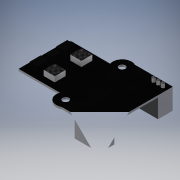
# Autodesk Inventor part: Encoder
Saved by Autodesk Inventor 2016 (Build 200138000, 138)
## iProperties
Created: 2017-02-27
Part Number: Encoder
Material: Generic
Document SubType Name: Modeling
Designer: jorge
Density: 1 g/cm^3
Appearance: Gray
Author: jorge
Autodesk Inventor part; units mm, degrees
note: some values were not read from the file. Chosen so that the rebuilt part matches the saved one: sketch regions of "Extrusion1".
ref_plane "YZ Plane" through (0, 0, 0) normal (1, 0, 0) x (0, 1, 0)
ref_plane "XZ Plane" through (0, 0, 0) normal (0, 1, 0) x (-1, 0, 0)
ref_plane "XY Plane" through (0, 0, 0) normal (0, 0, 1) x (1, 0, 0)
sketch "Sketch1" plane through (0, 0, 0) normal (0, 1, 0) x (-1, 0, 0)
  line L0 (0, 0) -> (0, -16)
  line L1 (0, -16) -> (-13, -16)
  circle A0 centre (48.4003, -12.7173) radius 1 projected
  circle A1 centre (48.4003, 5.2827) radius 1 projected
  line L2 (0, 0) -> (-13, 0)
  line L3 (-16, 0) -> (-16, 1.0033)
  line L4 (-16, -16) -> (-16, -17.0033)
  circle A2 centre (-16, 1.0033) radius 1
  circle A3 centre (-16, -17.0033) radius 1
  arc A4 (-18.8273, -16) -> (-13.1727, -16) centre (-16, -17.0033) ccw
  arc A5 (-13.1727, 0) -> (-18.8273, 0) centre (-16, 1.0033) ccw
  line L5 (-19, 0) -> (-29.5, 0)
  line L6 (-19, -16) -> (-29.5, -16)
  line L7 (-29.5, 0) -> (-29.5, -16)
  line L8 (-29.5, -8) -> (-29.5, -19.65)
  line L9 (-29.5, -8) -> (-29.5, 3.6592)
  line L10 (-29.5, 3.6592) -> (-17.3951, 3.6592)
  line L11 (-29.5, -19.65) -> (-17.4124, -19.65)
  line L12 (-13, 0) -> (-13.1727, 0)
  line L13 (-18.8273, 0) -> (-19, 0)
  line L14 (-13, -16) -> (-13.1727, -16)
  line L15 (-18.8273, -16) -> (-19, -16)
  dimension "d0" = 16
  dimension "d1" = 13
  dimension "d2" = 6
  dimension "d3" = 1.0033
  dimension "d4" = 1.0033
  dimension "d5" = 2
  dimension "d6" = 2
  dimension "d7" = 6
  dimension "d8" = 6
  dimension "d9" = 6
  dimension "d10" = 13
  dimension "d11" = 10.5
  dimension "d12" = 11.65
  constraints: 32 end point, 6 horizontal, 6 point on circle, 5 vertical, 4 centre point, 4 coincident, 2 point on line, 1 midpoint, 1 parallel, 1 perpendicular
  measures "d0" distance of L0.start L0.end
  measures "d1" distance of L0.end L1.end
  measures "d2" distance of L2.end L5.start
  measures "d3" distance of L3.start L3.end
  measures "d4" distance of L4.start L4.end
  measures "d5" diameter of A2
  measures "d6" diameter of A3
  measures "d7" diameter of A4
  measures "d8" diameter of A5
  measures "d9" distance of L1.end L6.start
  measures "d10" distance of L0.start L2.end
  measures "d11" distance of L5.start L5.end
  measures "d12" distance of L8.start L8.end
extrude "Extrusion1" add sketch "Sketch1" along normal blind 0.65 contours L0 L1 L14 A4 L15 L6 L7 L5 L13 A5 L12 L2 | A5 L13 L5 L9 L10 | L11 L8 L6 L15 A4
sketch "Sketch2" plane through (0, 0.65, 0) normal (0, 1, 0) x (1, 0, 0)
  line L0 (0, 0) -> (13.1727, 0) projected
  circle A0 centre (16, -1.0033) radius 1 projected
  circle A1 centre (16, 17.0033) radius 1 projected
  line L1 (17.3951, -3.6592) -> (29.5, -3.6592) projected
  line L2 (29.5, -3.6592) -> (29.5, 19.65) projected
  line L3 (29.5, 19.65) -> (17.4124, 19.65) projected
  arc A2 (17.4124, 19.65) -> (13.1727, 16) centre (16, 17.0033) ccw projected
  line L4 (13.1727, 16) -> (0, 16) projected
  line L5 (0, 16) -> (0, 0) projected
  line L6 (0, 0) -> (13.1727, 0) projected
  arc A3 (13.1727, 0) -> (17.3951, -3.6592) centre (16, -1.0033) ccw projected
  line L7 (0, 0) -> (1.5, 0)
  line L8 (1.5, 0) -> (1.5, 2)
  line L9 (1.5, 2) -> (0, 2)
  line L10 (0, 2) -> (0, 0)
  line L11 (1.5, 2) -> (4, 2)
  line L12 (4, 2) -> (4, 5.5)
  line L13 (4, 5.5) -> (1.5, 5.5)
  line L14 (1.5, 5.5) -> (1.5, 2)
  line L15 (4, 2) -> (6, 2)
  line L16 (4, 2) -> (6, 2) construction
  line L17 (6, 2) -> (6, 5.5)
  line L18 (6, 5.5) -> (9.5052, 5.5)
  line L19 (6, 2) -> (9.5052, 2)
  line L20 (9.5052, 2) -> (9.5052, 5.5)
  line L21 (9.5052, 5.5) -> (6, 5.5)
  line L22 (6, 5.5) -> (6, 2)
  circle A4 centre (28.0254, -2.0033) radius 0.5
  circle A5 centre (26.5254, -2.0033) radius 0.5
  line L23 (26.5254, -2.0033) -> (28.0254, -2.0033)
  line L24 (26.5254, -2.0033) -> (25.0254, -2.0033)
  circle A6 centre (25.0254, -2.0033) radius 0.5
  line L25 (29.5, 7.9954) -> (27.2754, 7.9954)
  line L26 (1.5, 15.9908) -> (1.5, 13.9908)
  line L27 (1.5, 13.9908) -> (0, 13.9908)
  line L28 (1.5, 13.9908) -> (4, 13.9908)
  line L29 (4, 13.9908) -> (4, 10.4908)
  line L30 (4, 10.4908) -> (1.5, 10.4908)
  line L31 (1.5, 10.4908) -> (1.5, 13.9908)
  line L32 (4, 13.9908) -> (6, 13.9908)
  line L33 (4, 13.9908) -> (6, 13.9908) construction
  line L34 (6, 13.9908) -> (6, 10.4908)
  line L35 (6, 10.4908) -> (9.5052, 10.4908)
  line L36 (6, 13.9908) -> (9.5052, 13.9908)
  line L37 (9.5052, 13.9908) -> (9.5052, 10.4908)
  line L38 (9.5052, 10.4908) -> (6, 10.4908)
  line L39 (6, 10.4908) -> (6, 13.9908)
  circle A7 centre (28.0254, 17.9941) radius 0.5
  circle A8 centre (26.5254, 17.9941) radius 0.5
  line L40 (26.5254, 17.9941) -> (28.0254, 17.9941)
  line L41 (26.5254, 17.9941) -> (25.0254, 17.9941)
  circle A9 centre (25.0254, 17.9941) radius 0.5
  line L42 (1.893, 6.5402) -> (3.725, 6.5402)
  line L43 (3.725, 6.5402) -> (3.725, 9.4507)
  line L44 (3.725, 9.4507) -> (1.893, 9.4507)
  line L45 (1.893, 9.4507) -> (1.893, 6.5402)
  dimension "d15" = 1.5
  dimension "d16" = 2
  dimension "d17" = 2.5
  dimension "d18" = 3.5
  dimension "d19" = 2
  dimension "d20" = 0
  dimension "d21" = 3.5052
  dimension "d22" = 90
  dimension "d23" = 1
  dimension "d24" = 1
  dimension "d25" = 1.5
  dimension "d26" = 1.5
  dimension "d27" = 1
  dimension "d33" = 1.0402
  dimension "d34" = 1.0402
  constraints: 78 end point, 16 symmetric about line, 9 horizontal, 8 parallel, 6 centre point, 6 perpendicular, 2 coincident, 1 collinear, 1 midpoint, 3 other
  measures "d15" distance of L9.end L8.end
  measures "d16" distance of L8.end L7.end
  measures "d17" distance of L13.end L12.end
  measures "d18" distance of L12.end L11.end
  measures "d19" distance of L11.end L15.end
  measures "d20" distance between parallel lines of L15 L16
  measures "d21" distance of L17.end L18.end
  measures "d22" angle of L17 L18
  measures "d23" diameter of A4
  measures "d24" diameter of A5
  measures "d25" distance of L23.start L23.end
  measures "d26" distance of L23.start L24.end
  measures "d27" diameter of A6
  measures "d33" distance between parallel lines of L30 L44
  measures "d34" distance between parallel lines of L13 L42
extrude "Extrusion2" add sketch "Sketch2" along normal blind 1.7 contours L14 L13 L12 L11 | L17 L18 L20 L19 | A4 | L23 L24 A5 | A5 L24 L23 | A6 | L28 L29 L30 L31 | L36 L37 L35 L34 | A7 | L40 L41 A8 | A8 L41 L40 | A9 | L45 L44 L43 L42
chamfer "Chamfer1" distance 0.5 angle 45 6 edges at (27.5254, 2.35, -17.9941) (26.0254, 2.35, -17.9941) (24.5254, 2.35, -17.9941) (27.5254, 2.35, 2.0033) (26.0254, 2.35, 2.0033) (24.5254, 2.35, 2.0033)
sketch "Sketch3" plane through (0, 0, 0) normal (0, -1, 0) x (1, 0, 0)
  circle A0 centre (16, -17.0033) radius 1 projected
  circle A1 centre (16, 1.0033) radius 1 projected
  line L0 (29.5, 3.6592) -> (29.5, -19.65) projected
  line L1 (17.3951, 3.6592) -> (29.5, 3.6592) projected
  arc A2 (17.3951, 3.6592) -> (13.1727, 0) centre (16, 1.0033) ccw projected
  line L2 (0, 0) -> (13.1727, 0) projected
  line L3 (0, -16) -> (0, 0) projected
  line L4 (13.1727, -16) -> (0, -16) projected
  arc A3 (13.1727, -16) -> (17.4124, -19.65) centre (16, -17.0033) ccw projected
  line L5 (29.5, -19.65) -> (17.4124, -19.65) projected
  line L6 (0, -16) -> (8, -16)
  line L7 (8, -16) -> (8, -11.3)
  line L8 (8, -11.3) -> (0, -11.3)
  line L9 (0, -11.3) -> (0, -16)
  line L10 (0, -16) -> (0, 0) projected
  line L11 (0, -8) -> (1.7097, -8)
  line L12 (0, 0) -> (0, -16)
  line L13 (13.1727, 0) -> (0, 0)
  line L14 (0, 0) -> (8, 0)
  line L15 (8, 0) -> (8, -4.7)
  line L16 (8, -4.7) -> (0, -4.7)
  line L17 (0, -4.7) -> (0, 0)
  line L18 (0, 0) -> (0, -16)
  line L19 (29.5, 3.6592) -> (29.5, -19.65) projected
  line L20 (29.5, -19.65) -> (21.5, -19.65)
  line L21 (21.5, -19.65) -> (21.5, -14.95)
  line L22 (21.5, -14.95) -> (29.5, -14.95)
  line L23 (29.5, -14.95) -> (29.5, -19.65)
  line L24 (29.5, 3.6592) -> (21.5, 3.6592)
  line L25 (21.5, 3.6592) -> (21.5, -1.0408)
  line L26 (21.5, -1.0408) -> (29.5, -1.0408)
  line L27 (29.5, -1.0408) -> (29.5, 3.6592)
  dimension "d35" = 8
  dimension "d36" = 4.7
  dimension "d39" = 8
  dimension "d40" = 4.7
  dimension "d41" = 8
  dimension "d42" = 4.7
  constraints: 40 end point, 6 parallel, 6 symmetric about line, 4 horizontal, 3 perpendicular, 1 midpoint
  measures "d35" distance of L8.end L7.end
  measures "d36" distance of L7.end L6.end
  measures "d39" distance of L21.end L22.end
  measures "d40" distance of L20.end L21.end
  measures "d41" distance of L26.end L25.end
  measures "d42" distance of L25.end L24.end
extrude "Extrusion3" add sketch "Sketch3" along normal blind 6 contours L0 L26 L25 L1 | L0 L5 L21 L22
equation "\"d34\" = d33"
body "Solid1"
